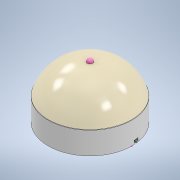
# Autodesk Inventor part: tutte
Saved by Autodesk Inventor 2020 (Build 240168000, 168)
## iProperties
Created: 2020-03-24
Part Number: tutte
Material: Generic
Document SubType Name: Modeling
Designer: magnu
Density: 1 g/cm^3
Appearance: Default
Mass: 25.2709 g
Surface Area: 257.936 cm^2
Volume: 25.2709 cm^3
Author: magnu
Autodesk Inventor part; units mm, degrees
sketch "Sketch1" plane through (0, 0, 0) normal (1, 0, 0) x (0, 1, 0)
  line L0 (50, 0) -> (0, 0)
  line L1 (0, 0) -> (0, -40)
  line L2 (0, -40) -> (21.3247, -40)
  line L3 (50, 0) -> (50, -2.7021)
  arc A0 (21.8707, -39.924) -> (50, -2.7021) centre (11.3084, -2.7021) ccw
  arc A1 (21.3247, -40) -> (21.8707, -39.924) centre (21.3247, -38) ccw
  point P0 (21.5993, -40)
  dimension "d0" = 40
  dimension "d1" = 50
  dimension "d2" = 2
  constraints: 8 end point, 5 point on circle, 3 tangent, 2 centre point, 2 horizontal, 1 perpendicular, 1 point on line, 1 vertical
  measures "d0" distance of L0.end L1.end
  measures "d1" distance of L0.start L0.end
  measures "d2" radius of A1
revolve "Revolution1" add sketch "Sketch1" angle 360 about axis through (0, 50, 0) along (0, -1, 0)
shell "Shell1" thickness 2 removed faces 1 at (-8.2294, 0, 6.0893)
ref_plane "Work Plane1" through (-40, 10.6624, 0) normal (1, 0, 0) x (0, 1, 0)
sketch "Sketch2" plane through (-40, 10.6624, 0) normal (1, 0, 0) x (0, 1, 0)
  line L0 (-10.6624, 40) -> (-10.6624, -40) projected
  line L1 (-10.6624, -4.4277) -> (-7.1624, -4.4277)
  line L2 (-7.1624, -4.4277) -> (-7.1624, -2.0547)
  line L3 (-9.3624, -2.2277) -> (-10.6624, -2.2277)
  line L4 (-10.6624, -2.2277) -> (-10.6624, -4.4277)
  line L5 (-9.3624, -2.2277) -> (-9.3624, -0.2277)
  line L6 (-7.1624, -0.2277) -> (-7.1624, -2.0547)
  line L7 (-7.1624, -0.2277) -> (-9.3624, -0.2277)
  point P0 (-10.6624, 0)
  dimension "d5" = 3.5
  dimension "d6" = 1.3
  dimension "d7" = 2
  dimension "d8" = 2.2
  constraints: 14 end point, 3 parallel, 2 horizontal, 1 perpendicular, 1 point on line
  measures "d5" distance of L1.start L1.end
  measures "d6" distance between parallel lines of L5 L0
  measures "d7" distance of L3.start L5.end
  measures "d8" distance between parallel lines of L1 L3
extrude "Extrusion1" cut sketch "Sketch2" along normal up to surface
sketch "Sketch4" plane through (0, 0, 0) normal (1, 0, 0) x (0, 1, 0)
  line L0 (50, 2.7021) -> (50, -2.7021) projected
  arc A0 (52.9601, 0) -> (50, 2.7021) centre (50.2468, 0) ccw
  line L1 (52.9601, 0) -> (50, 0)
  line L2 (-10.7112, 0) -> (64.2673, 0) projected
  point P0 (0, 0)
  constraints: 2 end point, 2 point on circle, 1 centre point, 1 midpoint
revolve "Revolution2" add sketch "Sketch4" angle 360 about axis through (0, -10, 0) along (0, 1, 0)
ref_plane "Work Plane2" through (0, 0, -0.1139) normal (0, 0, 1) x (1, 0, 0)
ref_plane "Work Plane5" through (40, 10.6624, 0) normal (1, 0, 0) x (0, 1, 0)
sketch "Sketch5" plane through (40, 10.6624, 0) normal (1, 0, 0) x (0, 1, 0)
  point P0 (-10.6624, 0)
ref_plane "Work Plane4" through (0, 0, -2.2139) normal (0, 0, 1) x (1, 0, 0)
ref_plane "Work Plane6" through (-38.7477, 0, -4.4277) normal (0, 0, 1) x (1, 0, 0)
ref_plane "Work Plane7" through (-37.9346, 0.65, -2.2277) normal (0, 0, 1) x (1, 0, 0)
sketch "Sketch7" plane through (40, 10.6624, 0) normal (1, 0, 0) x (0, 1, 0)
  line L0 (-10.6624, -2.2277) -> (-9.3624, -2.2277) projected
  line L1 (-10.6624, -2.2277) -> (-7.1624, -2.2277)
  line L2 (-7.1624, -2.2277) -> (-7.1624, -6.4277)
  line L3 (-7.1624, -6.4277) -> (-9.3624, -6.4277)
  line L4 (-9.3624, -6.4277) -> (-9.3624, -4.4277)
  line L5 (-10.6624, -4.4277) -> (-7.1624, -4.4277) projected
  line L6 (-10.6624, -4.4277) -> (-10.6624, -2.2277)
  line L7 (-10.6624, 40) -> (-10.6624, -40) projected
  point P0 (-10.6624, 0)
  dimension "d35" = 3.5
  dimension "d36" = 1.3
  constraints: 10 end point, 2 perpendicular, 1 horizontal, 1 parallel, 1 point on line, 1 vertical
  measures "d35" distance of L0.start L1.end
  measures "d36" distance between parallel lines of L7 L4
extrude "Extrusion4" cut sketch "Sketch7" against normal up to next
body "Solid1"
